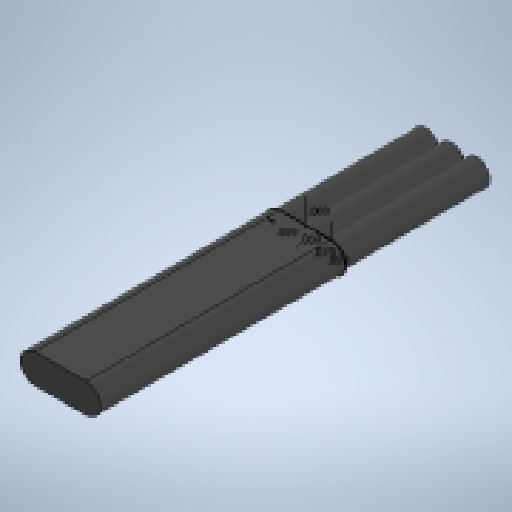
# Autodesk Inventor part: Cable Sleeve
Saved by Autodesk Inventor 2023.2 (Build 272271000, 271)
## iProperties
Created: 2024-02-01
Part Number: Cable Sleeve
Material: Rubber, Silicone
Document SubType Name: Modeling
Designer: Nathan Cai
Density: 1.25 g/cm^3
Appearance: Rubber - Black
Author: Nathan Cai
Autodesk Inventor part; units mm, degrees
ref_plane "YZ Plane" through (0, 0, 0) normal (1, 0, 0) x (0, 1, 0)
ref_plane "XZ Plane" through (0, 0, 0) normal (0, 1, 0) x (-1, 0, 0)
ref_plane "XY Plane" through (0, 0, 0) normal (0, 0, 1) x (1, 0, 0)
sketch "Sketch1" plane through (0, 0, 0) normal (0, 0, 1) x (1, 0, 0)
  line L0 (-1.75, 0) -> (1.75, 0) construction
  line L1 (-1.75, -1) -> (1.75, -1)
  line L2 (1.75, 1) -> (-1.75, 1)
  arc A0 (-1.75, 1) -> (-1.75, -1) centre (-1.75, 0) ccw
  arc A1 (1.75, -1) -> (1.75, 1) centre (1.75, 0) ccw
  circle A2 centre (0, 0) radius 0.875
  circle A3 centre (1.75, 0) radius 0.875
  circle A4 centre (-1.75, 0) radius 0.875
  point P0 (-0.875, 0)
  point P1 (0.875, 0)
  dimension "d0" = 1.75
  dimension "d1" = 2
  dimension "d4" = 1.75
  dimension "d5" = 1.75
  dimension "d6" = 1.75
  constraints: 8 end point, 5 centre point, 4 point on circle, 4 tangent, 3 coincident, 1 horizontal, 1 midpoint, 1 parallel
  measures "d0" distance of point (0, 0) L0.end
  measures "d1" diameter of A1
  measures "d4" diameter of A2
  measures "d5" diameter of A3
  measures "d6" diameter of A4
extrude "Extrusion1" add sketch "Sketch1" along normal blind 16.75 contours A0 L2 A1 L1 | A2 | A4 | A3
extrude "Extrusion2" add sketch "Sketch1" against normal blind 10 contours A2 | A4 | A3
body "Solid1"
